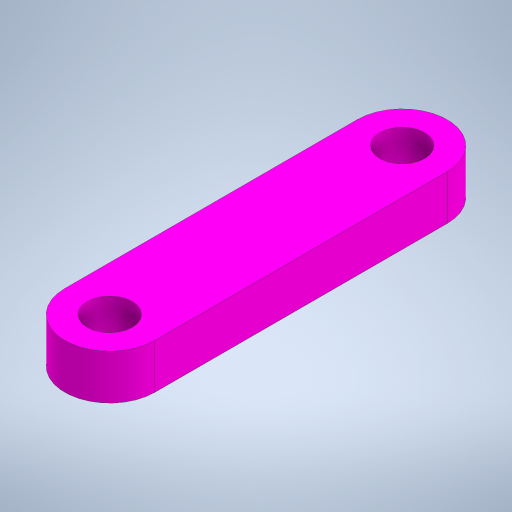
# Autodesk Inventor part: Base to Finger Connect
Saved by Autodesk Inventor 2023.1 (Build 271208000, 208)
## iProperties
Created: 2022-11-06
Part Number: Base to Finger Connect
Material: Generic
Document SubType Name: Modeling
Designer: shubh
Density: 1 g/cm^3
Appearance: Default
Author: shubh
Autodesk Inventor part; units mm, degrees
ref_plane "YZ Plane" through (0, 0, 0) normal (1, 0, 0) x (0, 1, 0)
ref_plane "XZ Plane" through (0, 0, 0) normal (0, 1, 0) x (-1, 0, 0)
ref_plane "XY Plane" through (0, 0, 0) normal (0, 0, 1) x (1, 0, 0)
sketch "Sketch1" plane through (0, 0, 0) normal (0, 1, 0) x (-1, 0, 0)
  circle A0 centre (0, 0) radius 3.175
  arc A1 (6.35, 0) -> (-6.35, 0) centre (0, 0) ccw
  circle A2 centre (0, -41.275) radius 3.175
  arc A3 (-6.35, -41.275) -> (6.35, -41.275) centre (0, -41.275) ccw
  line L0 (-6.35, -41.275) -> (-6.35, 0)
  line L1 (6.35, 0) -> (6.35, -41.275)
  point P0 (0, 0)
  point P1 (6.35, 0)
  dimension "d4" = 6.35
  dimension "d7" = 12.7
  dimension "d15" = 6.35
  dimension "d16" = 41.275
  dimension "d17" = 12.7
  constraints: 4 centre point, 4 end point, 4 point on circle, 3 coincident, 2 tangent, 1 parallel
  measures "d4" diameter of A0
  measures "d7" diameter of A1
  measures "d15" diameter of A2
  measures "d16" distance of point (0, 0) A2.centre
  measures "d17" diameter of A3
extrude "Extrusion1" add sketch "Sketch1" along normal blind 6.35
body "Solid1"
